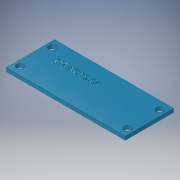
# Autodesk Inventor part: opencm9.04
Saved by Autodesk Inventor 2019 (Build 230136000, 136)
## iProperties
Created: 2020-11-08
Part Number: opencm9.04
Material: Типовые
Document SubType Name: Modeling
Designer: Петров Иван
Density: 1 g/cm^3
Appearance: Небесно-голубой
Author: Петров Иван
Autodesk Inventor part; units mm, degrees
ref_plane "YZ Plane" through (0, 0, 0) normal (1, 0, 0) x (0, 1, 0)
ref_plane "XZ Plane" through (0, 0, 0) normal (0, 1, 0) x (-1, 0, 0)
ref_plane "XY Plane" through (0, 0, 0) normal (0, 0, 1) x (1, 0, 0)
sketch "Эскиз1" plane through (0, 0, 0) normal (0, 1, 0) x (-1, 0, 0)
  line L0 (-33.25, 13.5) -> (33.25, 13.5)
  line L1 (33.25, 13.5) -> (33.25, -13.5)
  line L2 (33.25, -13.5) -> (-33.25, -13.5)
  line L3 (-33.25, -13.5) -> (-33.25, 13.5)
  line L4 (-33.25, 13.5) -> (33.25, -13.5) construction
  line L5 (33.25, 13.5) -> (-33.25, -13.5) construction
  point P0 (0, 0)
  dimension "d0" = 66.5
  dimension "d1" = 27
  constraints: 12 end point, 2 midpoint, 2 parallel, 1 horizontal, 1 perpendicular
  measures "d0" distance of L1.end L2.end
  measures "d1" distance of L0.end L1.end
extrude "Выдавливание1" add sketch "Эскиз1" along normal blind 2
sketch "Эскиз2" plane through (0, 2, 0) normal (0, 1, 0) x (1, 0, 0)
  circle A0 centre (-30, -9) radius 2
  circle A1 centre (30, -9) radius 2
  circle A2 centre (30, 9) radius 2
  circle A3 centre (-30, 9) radius 2
  line L0 (0, 0) -> (-7.0519, 0)
  line L1 (0, 0) -> (0, 8.4643)
  dimension "d4" = 4
  dimension "d5" = 4
  dimension "d6" = 4
  dimension "d7" = 4
  dimension "d9" = 9
  dimension "d10" = 30
  dimension "d11" = 30
  dimension "d12" = 30
  dimension "d13" = 9
  dimension "d14" = 9
  constraints: 4 centre point, 4 end point, 1 horizontal, 1 symmetric about line, 1 vertical
  measures "d4" diameter of A0
  measures "d5" diameter of A1
  measures "d6" diameter of A2
  measures "d7" diameter of A3
  measures "d9" vertical distance of L0.start A3.centre
  measures "d10" horizontal distance of L0.start A3.centre
  measures "d11" distance from line of L1 A1.centre
  measures "d12" distance from line of L1 A2.centre
  measures "d13" distance from line of L0 A1.centre
  measures "d14" distance from line of A2.centre L0
extrude "Выдавливание2" cut sketch "Эскиз2" against normal blind 2
sketch "Эскиз3" plane through (0, 2, 0) normal (0, 1, 0) x (1, 0, 0)
  line L0 (-23.2596, 5.7672) -> (20.3998, 5.7672) construction
  line L1 (20.3998, 5.7672) -> (20.3998, -6.9111) construction
  line L2 (20.3998, -6.9111) -> (-23.2596, -6.9111) construction
  line L3 (-23.2596, -6.9111) -> (-23.2596, 5.7672) construction
  spline S0 degree 2 poles (-20.7945, 5.3547) (-20.6216, 5.1522) (-20.4289, 4.5594) (-20.4289, 4.179) knots 0 0 0 1 2 2 2
  spline S1 degree 2 poles (-20.4289, 4.179) (-20.4289, 3.8085) (-20.6167, 3.2083) (-20.7945, 3.0058) knots 0 0 0 1 2 2 2
  spline S2 degree 2 poles (-20.7945, 3.0058) (-20.9822, 2.7933) (-21.4787, 2.5908) (-21.7776, 2.5908) knots 0 0 0 1 2 2 2
  spline S3 degree 2 poles (-21.7776, 2.5908) (-22.0863, 2.5908) (-22.5803, 2.8007) (-22.7606, 3.0058) knots 0 0 0 1 2 2 2
  spline S4 degree 2 poles (-22.7606, 3.0058) (-22.936, 3.2083) (-23.1237, 3.8036) (-23.1237, 4.179) knots 0 0 0 1 2 2 2
  spline S5 degree 2 poles (-23.1237, 4.179) (-23.1237, 4.5619) (-22.9335, 5.1448) (-22.7582, 5.3547) knots 0 0 0 1 2 2 2
  spline S6 degree 2 poles (-22.7582, 5.3547) (-22.5803, 5.5573) (-22.0839, 5.7672) (-21.7776, 5.7672) knots 0 0 0 1 2 2 2
  spline S7 degree 2 poles (-21.7776, 5.7672) (-21.4664, 5.7672) (-20.9674, 5.5499) (-20.7945, 5.3547) knots 0 0 0 1 2 2 2
  spline S8 degree 2 poles (-20.8513, 4.179) (-20.8513, 4.4804) (-20.9822, 4.9472) (-21.1008, 5.1003) knots 0 0 0 1 2 2 2
  spline S9 degree 2 poles (-21.1008, 5.1003) (-21.2218, 5.2584) (-21.5627, 5.4165) (-21.7751, 5.4165) knots 0 0 0 1 2 2 2
  spline S10 degree 2 poles (-21.7751, 5.4165) (-21.9949, 5.4165) (-22.3259, 5.2633) (-22.4519, 5.1003) knots 0 0 0 1 2 2 2
  spline S11 degree 2 poles (-22.4519, 5.1003) (-22.5729, 4.9447) (-22.7014, 4.4754) (-22.7014, 4.179) knots 0 0 0 1 2 2 2
  spline S12 degree 2 poles (-22.7014, 4.179) (-22.7014, 3.5788) (-22.1975, 2.9415) (-21.7751, 2.9415) knots 0 0 0 1 2 2 2
  spline S13 degree 2 poles (-21.7751, 2.9415) (-21.3527, 2.9415) (-20.8513, 3.5788) (-20.8513, 4.179) knots 0 0 0 1 2 2 2
  spline S14 degree 2 poles (-18.0577, 4.7842) (-18.0577, 4.5866) (-18.1985, 4.2309) (-18.3245, 4.1074) knots 0 0 0 1 2 2 2
  spline S15 degree 2 poles (-18.3245, 4.1074) (-18.4826, 3.9518) (-18.9099, 3.7912) (-19.2359, 3.7912) knots 0 0 0 1 2 2 2
  line L4 (-19.2359, 3.7912) -> (-19.5793, 3.7912)
  line L5 (-19.5793, 3.7912) -> (-19.5793, 2.655)
  line L6 (-19.5793, 2.655) -> (-19.9843, 2.655)
  line L7 (-19.9843, 2.655) -> (-19.9843, 5.703)
  line L8 (-19.9843, 5.703) -> (-19.2186, 5.703)
  spline S16 degree 2 poles (-19.2186, 5.703) (-18.9469, 5.703) (-18.5666, 5.6141) (-18.4208, 5.5128) knots 0 0 0 1 2 2 2
  spline S17 degree 2 poles (-18.4208, 5.5128) (-18.2504, 5.3967) (-18.0577, 5.0386) (-18.0577, 4.7842) knots 0 0 0 1 2 2 2
  spline S18 degree 2 poles (-18.4801, 4.7718) (-18.4801, 4.9299) (-18.5888, 5.1621) (-18.6999, 5.2362) knots 0 0 0 1 2 2 2
  spline S19 degree 2 poles (-18.6999, 5.2362) (-18.7963, 5.3004) (-19.0531, 5.3523) (-19.2433, 5.3523) knots 0 0 0 1 2 2 2
  line L9 (-19.2433, 5.3523) -> (-19.5793, 5.3523)
  line L10 (-19.5793, 5.3523) -> (-19.5793, 4.137)
  line L11 (-19.5793, 4.137) -> (-19.3026, 4.137)
  spline S20 degree 2 poles (-19.3026, 4.137) (-19.0556, 4.137) (-18.7518, 4.2161) (-18.653, 4.3198) knots 0 0 0 1 2 2 2
  spline S21 degree 2 poles (-18.653, 4.3198) (-18.5616, 4.4112) (-18.4801, 4.6261) (-18.4801, 4.7718) knots 0 0 0 1 2 2 2
  line L12 (-17.6724, 2.655) -> (-17.6724, 5.703)
  line L13 (-17.6724, 5.703) -> (-15.7656, 5.703)
  line L14 (-15.7656, 5.703) -> (-15.7656, 5.3424)
  line L15 (-15.7656, 5.3424) -> (-17.2673, 5.3424)
  line L16 (-17.2673, 5.3424) -> (-17.2673, 4.5075)
  line L17 (-17.2673, 4.5075) -> (-15.8668, 4.5075)
  line L18 (-15.8668, 4.5075) -> (-15.8668, 4.1469)
  line L19 (-15.8668, 4.1469) -> (-17.2673, 4.1469)
  line L20 (-17.2673, 4.1469) -> (-17.2673, 3.0156)
  line L21 (-17.2673, 3.0156) -> (-15.7656, 3.0156)
  line L22 (-15.7656, 3.0156) -> (-15.7656, 2.655)
  line L23 (-15.7656, 2.655) -> (-17.6724, 2.655)
  line L24 (-13.1399, 2.655) -> (-13.5944, 2.655)
  line L25 (-13.5944, 2.655) -> (-14.943, 5.2831)
  line L26 (-14.943, 5.2831) -> (-14.943, 2.655)
  line L27 (-14.943, 2.655) -> (-15.321, 2.655)
  line L28 (-15.321, 2.655) -> (-15.321, 5.703)
  line L29 (-15.321, 5.703) -> (-14.7454, 5.703)
  line L30 (-14.7454, 5.703) -> (-13.5178, 3.2898)
  line L31 (-13.5178, 3.2898) -> (-13.5178, 5.703)
  line L32 (-13.5178, 5.703) -> (-13.1399, 5.703)
  line L33 (-13.1399, 5.703) -> (-13.1399, 2.655)
  spline S22 degree 2 poles (-11.3319, 2.6007) (-11.6283, 2.6007) (-12.1297, 2.8007) (-12.3125, 3.0008) knots 0 0 0 1 2 2 2
  spline S23 degree 2 poles (-12.3125, 3.0008) (-12.4953, 3.1984) (-12.6953, 3.7912) (-12.6953, 4.1765) knots 0 0 0 1 2 2 2
  spline S24 degree 2 poles (-12.6953, 4.1765) (-12.6953, 4.5594) (-12.5002, 5.1275) (-12.3149, 5.3375) knots 0 0 0 1 2 2 2
  spline S25 degree 2 poles (-12.3149, 5.3375) (-12.1322, 5.5425) (-11.6332, 5.7574) (-11.3245, 5.7574) knots 0 0 0 1 2 2 2
  spline S26 degree 2 poles (-11.3245, 5.7574) (-11.1713, 5.7574) (-10.9021, 5.7129) (-10.7885, 5.6783) knots 0 0 0 1 2 2 2
  spline S27 degree 2 poles (-10.7885, 5.6783) (-10.6897, 5.6462) (-10.4847, 5.5548) (-10.3834, 5.5005) knots 0 0 0 1 2 2 2
  line L34 (-10.3834, 5.5005) -> (-10.3834, 5.0114)
  line L35 (-10.3834, 5.0114) -> (-10.4155, 5.0114)
  spline S28 degree 2 poles (-10.4155, 5.0114) (-10.4698, 5.0608) (-10.6378, 5.1991) (-10.7588, 5.2658) knots 0 0 0 1 2 2 2
  spline S29 degree 2 poles (-10.7588, 5.2658) (-10.8749, 5.33) (-11.1491, 5.4116) (-11.3269, 5.4116) knots 0 0 0 1 2 2 2
  spline S30 degree 2 poles (-11.3269, 5.4116) (-11.5221, 5.4116) (-11.8703, 5.251) (-12.0013, 5.0979) knots 0 0 0 1 2 2 2
  spline S31 degree 2 poles (-12.0013, 5.0979) (-12.1297, 4.9422) (-12.273, 4.4705) (-12.273, 4.1765) knots 0 0 0 1 2 2 2
  spline S32 degree 2 poles (-12.273, 4.1765) (-12.273, 3.8629) (-12.1223, 3.4108) (-11.9914, 3.2552) knots 0 0 0 1 2 2 2
  spline S33 degree 2 poles (-11.9914, 3.2552) (-11.8629, 3.1046) (-11.5196, 2.9514) (-11.3269, 2.9514) knots 0 0 0 1 2 2 2
  spline S34 degree 2 poles (-11.3269, 2.9514) (-11.1516, 2.9514) (-10.8527, 3.0379) (-10.7366, 3.1021) knots 0 0 0 1 2 2 2
  spline S35 degree 2 poles (-10.7366, 3.1021) (-10.6255, 3.1663) (-10.46, 3.2997) (-10.413, 3.3466) knots 0 0 0 1 2 2 2
  line L36 (-10.413, 3.3466) -> (-10.3834, 3.3466)
  line L37 (-10.3834, 3.3466) -> (-10.3834, 2.8625)
  spline S36 degree 2 poles (-10.3834, 2.8625) (-10.4847, 2.8156) (-10.6625, 2.7291) (-10.7885, 2.6896) knots 0 0 0 1 2 2 2
  spline S37 degree 2 poles (-10.7885, 2.6896) (-10.9219, 2.6451) (-11.1491, 2.6007) (-11.3319, 2.6007) knots 0 0 0 1 2 2 2
  line L38 (-7.3922, 2.655) -> (-7.7973, 2.655)
  line L39 (-7.7973, 2.655) -> (-7.7973, 5.2806)
  line L40 (-7.7973, 5.2806) -> (-8.5926, 3.4948)
  line L41 (-8.5926, 3.4948) -> (-8.8396, 3.4948)
  line L42 (-8.8396, 3.4948) -> (-9.6276, 5.2806)
  line L43 (-9.6276, 5.2806) -> (-9.6276, 2.655)
  line L44 (-9.6276, 2.655) -> (-10.0055, 2.655)
  line L45 (-10.0055, 2.655) -> (-10.0055, 5.703)
  line L46 (-10.0055, 5.703) -> (-9.4522, 5.703)
  line L47 (-9.4522, 5.703) -> (-8.6914, 4.0061)
  line L48 (-8.6914, 4.0061) -> (-7.9554, 5.703)
  line L49 (-7.9554, 5.703) -> (-7.3922, 5.703)
  line L50 (-7.3922, 5.703) -> (-7.3922, 2.655)
  spline S38 degree 2 poles (-6.9451, 4.7125) (-6.9451, 4.9472) (-6.792, 5.3375) (-6.6586, 5.4782) knots 0 0 0 1 2 2 2
  spline S39 degree 2 poles (-6.6586, 5.4782) (-6.5326, 5.6141) (-6.1646, 5.7648) (-5.9769, 5.7648) knots 0 0 0 1 2 2 2
  spline S40 degree 2 poles (-5.9769, 5.7648) (-5.7669, 5.7648) (-5.4261, 5.624) (-5.3001, 5.4906) knots 0 0 0 1 2 2 2
  spline S41 degree 2 poles (-5.3001, 5.4906) (-5.142, 5.3226) (-4.9691, 4.7792) (-4.9691, 4.3618) knots 0 0 0 1 2 2 2
  spline S42 degree 2 poles (-4.9691, 4.3618) (-4.9691, 3.9839) (-5.1395, 3.3071) (-5.305, 3.0823) knots 0 0 0 1 2 2 2
  spline S43 degree 2 poles (-5.305, 3.0823) (-5.4804, 2.8452) (-5.9744, 2.5957) (-6.335, 2.5957) knots 0 0 0 1 2 2 2
  spline S44 degree 2 poles (-6.335, 2.5957) (-6.4165, 2.5957) (-6.6018, 2.613) (-6.6808, 2.6377) knots 0 0 0 1 2 2 2
  line L51 (-6.6808, 2.6377) -> (-6.6808, 3.0305)
  line L52 (-6.6808, 3.0305) -> (-6.6611, 3.0305)
  spline S45 degree 2 poles (-6.6611, 3.0305) (-6.6092, 3.0008) (-6.3918, 2.9489) (-6.2807, 2.9489) knots 0 0 0 1 2 2 2
  spline S46 degree 2 poles (-6.2807, 2.9489) (-5.8806, 2.9489) (-5.4236, 3.4775) (-5.3915, 3.9666) knots 0 0 0 1 2 2 2
  spline S47 degree 2 poles (-5.3915, 3.9666) (-5.5545, 3.8554) (-5.8509, 3.7542) (-6.0263, 3.7542) knots 0 0 0 1 2 2 2
  spline S48 degree 2 poles (-6.0263, 3.7542) (-6.1942, 3.7542) (-6.4734, 3.8283) (-6.6141, 3.9345) knots 0 0 0 1 2 2 2
  spline S49 degree 2 poles (-6.6141, 3.9345) (-6.7772, 4.0605) (-6.9451, 4.4433) (-6.9451, 4.7125) knots 0 0 0 1 2 2 2
  spline S50 degree 2 poles (-5.3816, 4.4532) (-5.3816, 4.7619) (-5.4952, 5.1522) (-5.5965, 5.2584) knots 0 0 0 1 2 2 2
  spline S51 degree 2 poles (-5.5965, 5.2584) (-5.6854, 5.3572) (-5.8707, 5.4313) (-5.9794, 5.4313) knots 0 0 0 1 2 2 2
  spline S52 degree 2 poles (-5.9794, 5.4313) (-6.2313, 5.4313) (-6.5302, 5.0707) (-6.5302, 4.7298) knots 0 0 0 1 2 2 2
  spline S53 degree 2 poles (-6.5302, 4.7298) (-6.5302, 4.5372) (-6.4314, 4.2877) (-6.3227, 4.1988) knots 0 0 0 1 2 2 2
  spline S54 degree 2 poles (-6.3227, 4.1988) (-6.2436, 4.1346) (-6.0485, 4.0926) (-5.9349, 4.0926) knots 0 0 0 1 2 2 2
  spline S55 degree 2 poles (-5.9349, 4.0926) (-5.804, 4.0926) (-5.5026, 4.184) (-5.389, 4.2605) knots 0 0 0 1 2 2 2
  spline S56 degree 2 poles (-5.389, 4.2605) (-5.3865, 4.2902) (-5.3816, 4.3914) (-5.3816, 4.4532) knots 0 0 0 1 2 2 2
  line L53 (-3.9194, 2.655) -> (-4.4084, 2.655)
  line L54 (-4.4084, 2.655) -> (-4.4084, 3.2379)
  line L55 (-4.4084, 3.2379) -> (-3.9194, 3.2379)
  line L56 (-3.9194, 3.2379) -> (-3.9194, 2.655)
  spline S57 degree 2 poles (-1.4074, 4.179) (-1.4074, 3.359) (-1.8841, 2.5908) (-2.3805, 2.5908) knots 0 0 0 1 2 2 2
  spline S58 degree 2 poles (-2.3805, 2.5908) (-2.8844, 2.5908) (-3.3562, 3.3738) (-3.3562, 4.1765) knots 0 0 0 1 2 2 2
  spline S59 degree 2 poles (-3.3562, 4.1765) (-3.3562, 5.0015) (-2.8795, 5.7648) (-2.3805, 5.7648) knots 0 0 0 1 2 2 2
  spline S60 degree 2 poles (-2.3805, 5.7648) (-1.8791, 5.7648) (-1.4074, 4.9744) (-1.4074, 4.179) knots 0 0 0 1 2 2 2
  spline S61 degree 2 poles (-1.931, 3.2503) (-1.8717, 3.401) (-1.8223, 3.8653) (-1.8223, 4.179) knots 0 0 0 1 2 2 2
  spline S62 degree 2 poles (-1.8223, 4.179) (-1.8223, 4.4927) (-1.8717, 4.9546) (-1.9335, 5.1102) knots 0 0 0 1 2 2 2
  spline S63 degree 2 poles (-1.9335, 5.1102) (-1.9952, 5.2658) (-2.2101, 5.4264) (-2.3805, 5.4264) knots 0 0 0 1 2 2 2
  spline S64 degree 2 poles (-2.3805, 5.4264) (-2.551, 5.4264) (-2.7708, 5.2658) (-2.835, 5.1053) knots 0 0 0 1 2 2 2
  spline S65 degree 2 poles (-2.835, 5.1053) (-2.8968, 4.9497) (-2.9412, 4.4754) (-2.9412, 4.1765) knots 0 0 0 1 2 2 2
  spline S66 degree 2 poles (-2.9412, 4.1765) (-2.9412, 3.8554) (-2.9017, 3.4257) (-2.8375, 3.2577) knots 0 0 0 1 2 2 2
  spline S67 degree 2 poles (-2.8375, 3.2577) (-2.7782, 3.0996) (-2.5584, 2.9292) (-2.3805, 2.9292) knots 0 0 0 1 2 2 2
  spline S68 degree 2 poles (-2.3805, 2.9292) (-2.2126, 2.9292) (-1.9927, 3.0897) (-1.931, 3.2503) knots 0 0 0 1 2 2 2
  line L57 (0.9441, 3.7023) -> (0.581, 3.7023)
  line L58 (0.581, 3.7023) -> (0.581, 2.655)
  line L59 (0.581, 2.655) -> (0.1883, 2.655)
  line L60 (0.1883, 2.655) -> (0.1883, 3.7023)
  line L61 (0.1883, 3.7023) -> (-1.1579, 3.7023)
  line L62 (-1.1579, 3.7023) -> (-1.1579, 4.1321)
  line L63 (-1.1579, 4.1321) -> (0.2056, 5.703)
  line L64 (0.2056, 5.703) -> (0.581, 5.703)
  line L65 (0.581, 5.703) -> (0.581, 4.0308)
  line L66 (0.581, 4.0308) -> (0.9441, 4.0308)
  line L67 (0.9441, 4.0308) -> (0.9441, 3.7023)
  line L68 (0.1883, 4.0308) -> (0.1883, 5.2214)
  line L69 (0.1883, 5.2214) -> (-0.8368, 4.0308)
  line L70 (-0.8368, 4.0308) -> (0.1883, 4.0308)
  point P0 (0, 0)
  constraints: 2 other
extrude "Выдавливание3" cut sketch "Эскиз3" against normal blind 0.1
